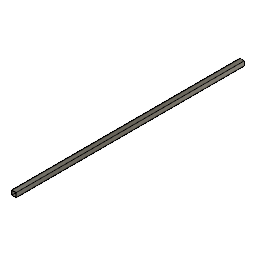
drone arm v2 (Autodesk Fusion 360 design; units mm, degrees)
Autodesk Fusion 360 part; units mm, degrees
sketch "Sketch1" plane through (0, 0, 0) normal (1, 0, 0) x (0, 1, 0)
  line L0 (-125, 0) -> (375, 0)
  dimension "d1" = 500
  constraint horizontal L0
  measures "d1" distance of L0.start L0.end
sketch "Sketch4" plane through (0, 0, 0) normal (0, 1, 0) x (1, 0, 0)
  line L0 (2.79, 7.645) -> (-7.71, 7.645)
  line L1 (-7.71, 7.645) -> (-7.71, -2.855)
  line L2 (-7.71, -2.855) -> (2.79, -2.855)
  line L3 (2.79, -2.855) -> (2.79, 7.645)
  line L4 (2.79, 7.645) -> (-7.71, -2.855) construction
  line L5 (-7.71, 7.645) -> (2.79, -2.855) construction
  line L6 (1.79, 6.645) -> (-6.71, 6.645)
  line L7 (-6.71, 6.645) -> (-6.71, -1.855)
  line L8 (-6.71, -1.855) -> (1.79, -1.855)
  line L9 (1.79, -1.855) -> (1.79, 6.645)
  line L10 (1.79, 6.645) -> (-6.71, -1.855) construction
  line L11 (-6.71, 6.645) -> (1.79, -1.855) construction
  point P0 (-2.46, 2.395)
  point P1 (-2.46, 2.395)
  dimension "d2" = 10.5
  dimension "d3" = 10.5
  dimension "d4" = 8.5
  dimension "d5" = 8.5
  constraint horizontal L0
  constraint perpendicular L0 L1
  constraint parallel L0 L2
  constraint parallel L1 L3
  constraint coincident L4 P1
  constraint coincident L5 P1
  constraint horizontal L6
  constraint perpendicular L6 L7
  constraint parallel L6 L8
  constraint parallel L7 L9
  constraint coincident L10 P1
  constraint coincident L11 P1
  constraint coincident P1 P0
  measures "d2" distance of L1.end L2.end
  measures "d3" distance of L0.end L1.end
  measures "d4" distance of L7.end L8.end
  measures "d5" distance of L6.end L7.end
sweep "Sweep1" add kept parallel profiles "Sketch4" path "Sketch1" along L0 section 1
